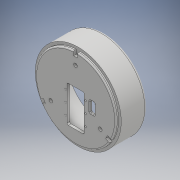
# Autodesk Inventor part: base_enclosure_1
Saved by Autodesk Inventor 2018 (Build 220112000, 112)
## iProperties
Created: 2018-04-10
Part Number: base_enclosure_1
Material: Generic
Document SubType Name: Modeling
Designer: mshaw2
Density: 1 g/cm^3
Appearance: Default
Author: mshaw2
## iProperties of the stored document base_enclosure_1_3DPrint.ipt
Created: 2018-04-18
Part Number: base_enclosure_1_3DPrint
Material: Generic
Document SubType Name: Modeling
Designer: mshaw2
Density: 1 g/cm^3
Appearance: Default
Author: mshaw2
Autodesk Inventor part; units mm, degrees
ref_plane "YZ Plane" through (0, 0, 0) normal (1, 0, 0) x (0, 1, 0)
ref_plane "XZ Plane" through (0, 0, 0) normal (0, 1, 0) x (-1, 0, 0)
ref_plane "XY Plane" through (0, 0, 0) normal (0, 0, 1) x (1, 0, 0)
sketch "Sketch1" plane through (0, 0, 0) normal (0, 1, 0) x (-1, 0, 0)
  arc A0 (-11.6454, 11.6645) -> (-12.2, 10.5) centre (-10.7, 10.5) ccw construction
  arc A1 (-11.6454, 11.6645) -> (-12.6157, 11.0765) centre (-11.3, 10) ccw construction
  line L0 (-12.6157, 11.0765) -> (-17.1157, 5.5765) construction
  arc A2 (-17.1157, 5.5765) -> (-17.5, 4.5) centre (-15.8, 4.5) ccw construction
  line L1 (-17.5, 4.5) -> (-17.5, -31.1) construction
  arc A3 (-17.5, -31.1) -> (-17.1157, -32.1765) centre (-15.8, -31.1) ccw construction
  line L2 (-17.1157, -32.1765) -> (-12.6157, -37.6765) construction
  arc A4 (-12.6157, -37.6765) -> (-11.3, -38.3) centre (-11.3, -36.6) ccw construction
  line L3 (-11.3, -38.3) -> (11.3, -38.3) construction
  arc A5 (11.3, -38.3) -> (12.6157, -37.6765) centre (11.3, -36.6) ccw construction
  line L4 (12.6157, -37.6765) -> (17.1157, -32.1765) construction
  arc A6 (17.1157, -32.1765) -> (17.5, -31.1) centre (15.8, -31.1) ccw construction
  line L5 (17.5, -31.1) -> (17.5, 4.5) construction
  arc A7 (17.5, 4.5) -> (17.1157, 5.5765) centre (15.8, 4.5) ccw construction
  line L6 (17.1157, 5.5765) -> (12.6157, 11.0765) construction
  arc A8 (12.6157, 11.0765) -> (11.6454, 11.6645) centre (11.3, 10) ccw construction
  arc A9 (12.2, 10.5) -> (11.6454, 11.6645) centre (10.7, 10.5) ccw construction
  line L7 (12.2, 10.5) -> (12.2, -31.5) construction
  arc A10 (10.7, -33) -> (12.2, -31.5) centre (10.7, -31.5) ccw construction
  line L8 (-10.7, -33) -> (10.7, -33) construction
  arc A11 (-12.2, -31.5) -> (-10.7, -33) centre (-10.7, -31.5) ccw construction
  line L9 (-12.2, 10.5) -> (-12.2, -31.5) construction
  circle A12 centre (-8.5, -35.8) radius 1.2 construction
  circle A13 centre (8.5, -35.8) radius 1.2 construction
  circle A14 centre (-15, 4.5) radius 1.2
  circle A15 centre (-15, -12.5) radius 1.2
  circle A16 centre (-15, -29.5) radius 1.2
  circle A17 centre (15, -29.5) radius 1.2
  circle A18 centre (15, -12.5) radius 1.2
  circle A19 centre (15, 4.5) radius 1.2
  line L10 (11.3, -38.6) -> (-11.3, -38.6) construction
  arc A20 (-12.8479, -37.8665) -> (-11.3, -38.6) centre (-11.3, -36.6) ccw construction
  line L11 (-12.8479, -37.8665) -> (-17.3479, -32.3665) construction
  arc A21 (-17.8, -31.1) -> (-17.3479, -32.3665) centre (-15.8, -31.1) ccw construction
  line L12 (-17.8, -31.1) -> (-17.8, 4.5) construction
  line L13 (17.3479, -32.3665) -> (12.8479, -37.8665) construction
  arc A22 (11.3, -38.6) -> (12.8479, -37.8665) centre (11.3, -36.6) ccw construction
  line L14 (17.8, 4.5) -> (17.8, -31.1) construction
  arc A23 (17.3479, -32.3665) -> (17.8, -31.1) centre (15.8, -31.1) ccw construction
  arc A24 (17.8, 4.5) -> (17.3479, 5.7665) centre (15.8, 4.5) ccw construction
  line L15 (12.8479, 11.2665) -> (17.3479, 5.7665) construction
  arc A25 (12.8479, 11.2665) -> (11.3, 12) centre (11.3, 10) ccw construction
  spline S0 degree 3 poles (11.3, 11.8748) (11.3318, 11.8609) (11.3649, 11.8451) (11.4851, 11.7818) (11.5689, 11.7267) (11.6454, 11.6645) knots -0.198467 -0.198467 -0.198467 -0.198467 -0.191756 -0.191756 -0.174636 -0.174636 -0.174636 -0.174636 construction
  spline S1 degree 3 poles (11.3, 11.8748) (11.2559, 11.894) (11.211, 11.9111) (11.0105, 11.9765) (10.8493, 12) (10.7, 12) knots -0.063423 -0.063423 -0.063423 -0.063423 -0.049053 -0.049053 0 0 0 0 construction
  arc A26 (-11.3, 12) -> (-12.8479, 11.2665) centre (-11.3, 10) ccw construction
  line L16 (-11.3, 12) -> (-10.7, 12) construction
  line L17 (-17.3479, 5.7665) -> (-12.8479, 11.2665) construction
  spline S2 degree 3 poles (-11.3, 11.8748) (-11.3932, 11.8341) (-11.4972, 11.777) (-11.6151, 11.6887) (-11.6305, 11.6767) (-11.6454, 11.6645) knots 0.037429 0.037429 0.037429 0.037429 0.058499 0.058499 0.061766 0.061766 0.061766 0.061766 construction
  spline S3 degree 3 poles (-10.7, 12) (-10.8493, 12) (-11.0105, 11.9765) (-11.211, 11.9111) (-11.2559, 11.894) (-11.3, 11.8748) knots -0.307639 -0.307639 -0.307639 -0.307639 -0.258586 -0.258586 -0.244216 -0.244216 -0.244216 -0.244216 construction
  line L18 (10.7, 12) -> (11.3, 12) construction
  arc A27 (-17.3479, 5.7665) -> (-17.8, 4.5) centre (-15.8, 4.5) ccw construction
  circle A28 centre (0, 0) radius 5 construction
  circle A29 centre (0, 0) radius 61
  circle A30 centre (0, 0) radius 51
  circle A31 centre (0, 0) radius 65
  line L19 (-13, 14.2) -> (13, 14.2)
  line L20 (13, 14.2) -> (13, -40.8)
  line L21 (13, -40.8) -> (-13, -40.8)
  line L22 (-13, -40.8) -> (-13, 14.2)
  line L23 (-13, 14.2) -> (13, -40.8) construction
  line L24 (13, 14.2) -> (-13, -40.8) construction
  point P0 (0, -13.3)
  dimension "d0" = 122
  dimension "d1" = 10
  dimension "d2" = 4
  dimension "d3" = 26
  dimension "d4" = 55
  constraints: 50 end point, 40 point on circle, 32 centre point, 6 horizontal, 6 vertical, 2 midpoint, 2 parallel, 1 coincident, 1 perpendicular, 122 other
  measures "d0" diameter of A29
  measures "d1" radial gap between concentric circles of A29 A30
  measures "d2" radial gap between concentric circles of A29 A31
  measures "d3" distance of L20.end L21.end
  measures "d4" distance of L19.end L20.end
extrude "Extrusion1" add sketch "Sketch1" along normal blind 35.5 contours A29
extrude "Extrusion2" add sketch "Sketch1" against normal blind 4 contours A29 | A30
extrude "Extrusion3" add sketch "Sketch1" along normal blind 39.5 contours A31
sketch "Sketch2" plane through (0, -4, 0) normal (0, -1, 0) x (1, 0, 0)
  line L0 (13, 14.2) -> (13, -40.8) construction
  line L1 (13, -40.8) -> (-13, -40.8) construction
  line L2 (-13, -40.8) -> (-13, 14.2) construction
  line L3 (-13, 14.2) -> (13, 14.2) construction
  circle A0 centre (-15, 4.5) radius 1.2 construction
  circle A1 centre (-15, -12.5) radius 1.2 construction
  circle A2 centre (-15, -29.5) radius 1.2 construction
  circle A3 centre (15, -29.5) radius 1.2 construction
  circle A4 centre (15, -12.5) radius 1.2 construction
  circle A5 centre (15, 4.5) radius 1.2 construction
  circle A6 centre (0, 0) radius 61 construction
  line L4 (-3, 54.2) -> (3, 54.2)
  line L5 (3, 54.2) -> (3, 60.9262)
  circle A7 centre (0, 0) radius 61 projected
  line L6 (-3, 54.2) -> (-3, 60.9262)
  line L7 (-13, 14.2) -> (13, 14.2) projected
  line L8 (-13, -40.8) -> (-13, 14.2) projected
  line L9 (13, 14.2) -> (13, -40.8) projected
  line L10 (0, 14.2) -> (0, 54.2) construction
  arc A8 (3, 60.9262) -> (-3, 60.9262) centre (0, 0) ccw
  dimension "d14" = 40
  dimension "d15" = 6
  constraints: 8 end point, 5 parallel, 4 point on circle, 2 midpoint, 1 centre point, 1 coincident, 1 vertical
  measures "d14" distance between parallel lines of L3 L4
  measures "d15" distance between parallel lines of L5 L6
extrude "Extrusion5" cut sketch "Sketch2" against normal up to surface (4 mm away) contours L6 A7 L5 L4 picked at (0.3335, 56.4639)
pattern_circular "Circular Pattern1" count 3 over 360 about axis through (0, 0, 0) along (0, 1, 0) of "Extrusion5"
sketch "Sketch3" plane through (0, 0, 0) normal (0, 1, 0) x (1, 0, 0)
  line L0 (28, 7.5) -> (22, 7.5)
  line L1 (22, 7.5) -> (22, -7.5)
  line L2 (22, -7.5) -> (28, -7.5)
  line L3 (28, -7.5) -> (28, 7.5)
  line L4 (28, 7.5) -> (22, -7.5) construction
  line L5 (22, 7.5) -> (28, -7.5) construction
  line L6 (13, 40.8) -> (13, -14.2) projected
  point P0 (0, 0)
  point P1 (25, 0)
  dimension "d21" = 6
  dimension "d22" = 15
  dimension "d23" = 9
  dimension "d24" = 40.8
  constraints: 12 end point, 2 midpoint, 2 parallel, 1 horizontal, 1 perpendicular
  measures "d21" distance of L2.end L1.end
  measures "d22" distance of L1.end L0.end
  measures "d23" distance between parallel lines of L1 L6
  measures "d24" vertical distance of L6.start point (25, 0)
extrude "Extrusion6" cut sketch "Sketch3" against normal through all
fillet "Fillet2" radius 1 4 edges at (28, -2, 7.5) (28, -2, -7.5) (22, -2, -7.5) (22, -2, 7.5)
fillet "Fillet3" radius 2 24 edges at (13, -2, -40.8) (13, -2, 14.2) (-13, -2, 14.2) (-13, -2, -40.8) (51, 0, 0) (52.8275, -4, 30.5) (-52.8275, -4, 30.5) (0, -4, -61) (22.2929, 0, -7.2071) (25, 0, -7.5) (27.7071, 0, -7.2071) (28, 0, 0) (27.7071, 0, 7.2071) (25, 0, 7.5) (22.2929, 0, 7.2071) (22, 0, 0) (22.2929, -4, 7.2071) (25, -4, 7.5) (27.7071, -4, 7.2071) (28, -4, 0) (27.7071, -4, -7.2071) (25, -4, -7.5) (22.2929, -4, -7.2071) (22, -4, 0)
fillet "Fillet4" radius 4 1 edges at (65, 39.5, 0)
sketch "Sketch7" plane through (0, -4, 0) normal (0, -1, 0) x (1, 0, 0)
  line L0 (3, 54.2) -> (-3, 54.2) projected
  point P0 (0, 0)
  point P1 (0, 43.2)
  dimension "d33" = 11
  measures "d33" distance from line of L0 point (0, 43.2)
hole "Hole1" at (0, -4, 43.2) direction (0, 1, 0) diameter 5.5 depth 8 tip angle 118
pattern_circular "Circular Pattern2" count 3 over 360 about axis through (0, 0, 0) along (0, 1, 0) of "Hole1"
body "Solid1"
